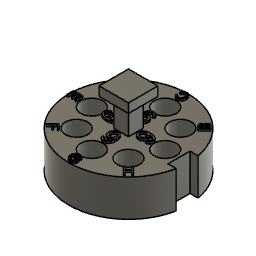
gasChargingBombHolderCryologgerstand v5 (Autodesk Fusion 360 design; units mm, degrees)
Autodesk Fusion 360 part; units mm, degrees
sketch "Skizze1" plane through (0, 0, 0) normal (0, 1, 0) x (1, 0, 0)
  circle A0 centre (0, 0) radius 32.5
  dimension "d1" = 65
  constraint coincident A0.centre origin
  measures "d1" diameter of A0
extrude "Extrusion1" add sketch "Skizze1" along normal blind 20 makes body 1
sketch "Skizze2" plane through (0, 20, 0) normal (0, 1, 0) x (-1, 0, 0)
  circle A0 centre (0, 0) radius 32.5
  circle A1 centre (20, 0) radius 6
  circle A2 centre (14.1421, 14.1421) radius 6
  circle A3 centre (0, 20) radius 6
  circle A4 centre (-14.1421, 14.1421) radius 6
  circle A5 centre (-20, 0) radius 6
  circle A6 centre (-14.1421, -14.1421) radius 6
  circle A7 centre (0, -20) radius 6
  circle A8 centre (14.1421, -14.1421) radius 6
  line L0 (4, -4) -> (-4, -4)
  line L1 (-4, -4) -> (-4, 4)
  line L2 (-4, 4) -> (4, 4)
  line L3 (4, 4) -> (4, -4)
  line L4 (4, -4) -> (-4, 4) construction
  line L5 (-4, -4) -> (4, 4) construction
  line L6 (40, 0) -> (-40, 0) construction
  line L7 (32.5, -2.75) -> (32.5, 2.75) construction
  line L8 (32.5, 2.75) -> (26, 2.75) construction
  line L9 (26, 2.75) -> (26, -2.75) construction
  line L10 (26, -2.75) -> (32.5, -2.75) construction
  line L11 (-21.0364, 24.9255) -> (-24.9255, 21.0364) construction
  line L12 (-24.9255, 21.0364) -> (-20.3293, 16.4402) construction
  line L13 (-20.3293, 16.4402) -> (-16.4402, 20.3293) construction
  line L14 (-16.4402, 20.3293) -> (-21.0364, 24.9255) construction
  line L15 (24.928, 21.034) -> (21.034, 24.928) construction
  line L16 (21.034, 24.928) -> (16.4378, 20.3318) construction
  line L17 (16.4378, 20.3318) -> (20.3318, 16.4378) construction
  line L18 (20.3318, 16.4378) -> (24.928, 21.034) construction
  line L19 (2.75, 32.5) -> (-2.75, 32.5) construction
  line L20 (-2.75, 32.5) -> (-2.75, 26) construction
  line L21 (-2.75, 26) -> (2.75, 26) construction
  line L22 (2.75, 26) -> (2.75, 32.5) construction
  line L23 (-5.1647, -32.5) -> (5.1647, -32.5) construction
  line L24 (5.1647, -32.5) -> (5.1647, -26) construction
  line L25 (5.1647, -26) -> (-5.1647, -26) construction
  line L26 (-5.1647, -26) -> (-5.1647, -32.5) construction
  line L27 (-26.3734, -19.5886) -> (-19.5886, -26.3734) construction
  line L28 (-19.5886, -26.3734) -> (-14.9924, -21.7772) construction
  line L29 (-14.9924, -21.7772) -> (-21.7772, -14.9924) construction
  line L30 (-21.7772, -14.9924) -> (-26.3734, -19.5886) construction
  line L31 (20.959, -25.0029) -> (25.0029, -20.959) construction
  line L32 (25.0029, -20.959) -> (20.4067, -16.3629) construction
  line L33 (20.4067, -16.3629) -> (16.3629, -20.4067) construction
  line L34 (16.3629, -20.4067) -> (20.959, -25.0029) construction
  circle A9 centre (0, 0) radius 5 construction
  line L35 (14, -5.0131) -> (14, 5.0131) construction
  line L36 (14, 5.0131) -> (5, 5.0131) construction
  line L37 (5, 5.0131) -> (5, -5.0131) construction
  line L38 (5, -5.0131) -> (14, -5.0131) construction
  line L39 (-5.0131, -14) -> (5.0131, -14) construction
  line L40 (5.0131, -14) -> (5.0131, -5) construction
  line L41 (5.0131, -5) -> (-5.0131, -5) construction
  line L42 (-5.0131, -5) -> (-5.0131, -14) construction
  line L43 (-14, 5.0131) -> (-14, -5.0131) construction
  line L44 (-14, -5.0131) -> (-5, -5.0131) construction
  line L45 (-5, -5.0131) -> (-5, 5.0131) construction
  line L46 (-5, 5.0131) -> (-14, 5.0131) construction
  line L47 (5.0131, 14) -> (-5.0131, 14) construction
  line L48 (-5.0131, 14) -> (-5.0131, 5) construction
  line L49 (-5.0131, 5) -> (5.0131, 5) construction
  line L50 (5.0131, 5) -> (5.0131, 14) construction
  point P0 (32.5, 0)
  point P1 (22.981, 22.981)
  point P2 (0, 32.5)
  point P3 (-22.981, 22.981)
  point P4 (-32.5, 0)
  point P5 (-22.981, -22.981)
  point P6 (0, -32.5)
  point P7 (22.981, -22.981)
  point P8 (5, 0)
  point P9 (0, 5)
  point P10 (-5, 0)
  point P11 (0, -5)
  dimension "d5" = 12
  dimension "d6" = 20
  dimension "d13" = 360
  dimension "d23" = 8
  dimension "d24" = 8
  dimension "d34" = 360
  dimension "d35" = 5
  dimension "d37" = 5
  dimension "d39" = 5
  dimension "d40" = 5
  dimension "d41" = 5
  dimension "d42" = 5
  dimension "d43" = 5
  dimension "d44" = 10
  dimension "d45" = 8
  dimension "d46" = 8
  dimension "d47" = 8
  dimension "d48" = 8
  dimension "d50" = 360
  text T0 "E" font "Arial" height 5 align centre middle in box 5.5 x 6.5 at (32.5, -2.75) x (0, 1) y (-1, 0) spacing 1
  text T1 "H" font "Arial" height 5 align centre middle in box 5.5 x 6.5 at (-21.0364, 24.9255) x (-0.707107, -0.707107) y (0.707107, -0.707107) spacing 1
  text T2 "F" font "Arial" height 5 align centre middle in box 5.507 x 6.5 at (24.928, 21.034) x (-0.707107, 0.707106) y (-0.707106, -0.707107) spacing 1
  text T3 "G" font "Arial" height 5 align centre middle in box 5.5 x 6.5 at (2.75, 32.5) x (-1, 0) y (0, -1) spacing 1
  text T4 "C" font "Arial" height 5 align centre middle in box 10.3294 x 6.5 at (-5.1647, -32.5) x (1, 0) y (0, 1) spacing 1
  text T5 "B" font "Arial" height 5 align centre middle in box 9.5952 x 6.5 at (-26.3734, -19.5886) x (0.707106, -0.707107) y (0.707107, 0.707106) spacing 1
  text T6 "D" font "Arial" height 5 align centre middle in box 5.7189 x 6.5 at (20.959, -25.0029) x (0.707107, 0.707107) y (-0.707107, 0.707107) spacing 1
  text T7 "9" font "Arial" height 8 align centre middle in box 10.0261 x 9 at (14, -5.0131) x (0.000001, 1) y (-1, 0.000001) spacing 1
  text T8 "9" font "Arial" height 8 align centre middle in box 10.0261 x 9 at (-5.0131, -14) x (1, -0.000001) y (0.000001, 1) spacing 1
  text T9 "9" font "Arial" height 8 align centre middle in box 10.0261 x 9 at (-14, 5.0131) x (-0.000001, -1) y (1, -0.000001) spacing 1
  text T10 "9" font "Arial" height 8 align centre middle in box 10.0261 x 9 at (5.0131, 14) x (-1, 0.000001) y (-0.000001, -1) spacing 1
  constraint coincident A0.centre A9.centre
  constraint horizontal L0
  constraint perpendicular L0 L1
  constraint parallel L0 L2
  constraint parallel L1 L3
  constraint coincident L4 A0.centre
  constraint coincident L5 A0.centre
  constraint perpendicular L1 L6
  constraint coincident L6 P0
  constraint coincident A0 P0
  constraint coincident P0
  constraint coincident P7
  constraint tangent A0 L31
  constraint coincident A1
  constraint coincident A8
  constraint coincident P6
  constraint coincident A7
  constraint tangent A0 L23
  constraint coincident P5
  constraint coincident A6
  constraint tangent A0 L27
  constraint coincident P3
  constraint coincident A4
  constraint tangent A0 L11
  constraint coincident P2
  constraint coincident A3
  constraint tangent A0 L19
  constraint coincident P1
  constraint coincident A2
  constraint tangent A0 L15
  constraint concentric A0 A9
  constraint coincident L6 P8
  constraint coincident A9 P8
  constraint coincident P8
  constraint tangent A1 L35
  constraint coincident P9
  constraint tangent A3 L47
  constraint coincident P11
  constraint tangent A7 L39
  constraint coincident P10
  constraint tangent A5 L43
  measures "d5" diameter of A1
  measures "d6" distance of A0.centre A1.centre
  measures "d23" distance of L1.end L2.end
  measures "d24" distance of L0.end L1.end
  measures "d44" diameter of A9
extrude "Extrusion3" cut sketch "Skizze2" against normal blind 15 contours A1 | A2 | A3 | A4 | A5 | A6 | A7 | A8 bodies 1
extrude "Extrusion5" add sketch "Skizze2" along normal blind 15 contours L0 L1 L2 L3 bodies 1
ref_plane "Arbeitsebene1" through (0, 40, 0) normal (0, 1, 0) x (-1, 0, 0)
sketch "Skizze3" plane through (0, 40, 0) normal (0, 1, 0) x (1, 0, 0)
  line L0 (8, 8) -> (-8, 8)
  line L1 (-8, 8) -> (-8, -8)
  line L2 (-8, -8) -> (8, -8)
  line L3 (8, -8) -> (8, 8)
  line L4 (8, 8) -> (-8, -8) construction
  line L5 (-8, 8) -> (8, -8) construction
  constraint horizontal L0
  constraint perpendicular L0 L1
  constraint parallel L0 L2
  constraint parallel L1 L3
  constraint coincident L4 origin
  constraint coincident L5 origin
extrude "Extrusion6" add sketch "Skizze3" against normal blind 5 separate body makes body 2
ref_plane "Arbeitsebene2" through (32.5, 10.3248, 0) normal (1, 0, 0) x (0, 0, 1)
sketch "Skizze4" plane through (32.5, 0, 0) normal (1, 0, 0) x (0, 0, -1)
  line L0 (6, 20) -> (-6, 20)
  line L1 (-6, 20) -> (-6, 0)
  line L2 (-6, 0) -> (6, 0)
  line L3 (6, 0) -> (6, 20)
  line L4 (6, 20) -> (-6, 0) construction
  line L5 (-6, 20) -> (6, 0) construction
  point P0 (0, 10)
  constraint horizontal L0
  constraint perpendicular L0 L1
  constraint parallel L0 L2
  constraint parallel L1 L3
  constraint coincident L4 P0
  constraint coincident L5 P0
extrude "Extrusion7" cut sketch "Skizze4" against normal blind 5 bodies 1
extrude "Extrusion8" add sketch "Skizze2" along normal blind 1 text T1 T3 T2 T0 T4 T5 T9 T8 T7 T10 T6 bodies 1
